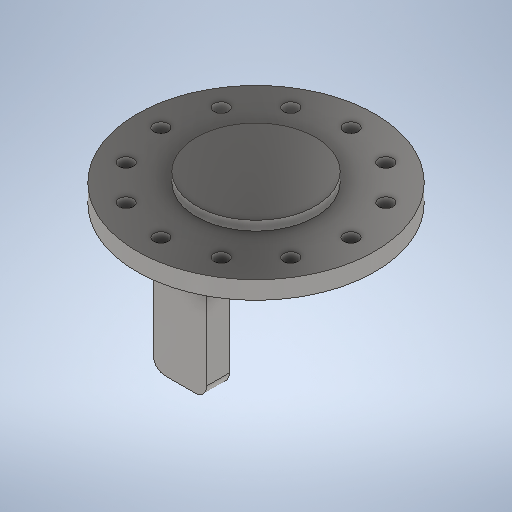
# Autodesk Inventor part: EndEffector
Saved by Autodesk Inventor 2025.1 (Build 291241000, 241)
## iProperties
Created: 2025-01-29
Part Number: EndEffector
Material: Steel, High Strength, Low Alloy
Document SubType Name: Modeling
Designer: yovan
Mass: 4767.32 g
Surface Area: 922.718 cm^2
Volume: 607.302 cm^3
Density: 7.85 g/cm^3
Appearance: Steel - Polished
Author: yovan
Autodesk Inventor part; units mm, degrees
ref_plane "YZ Plane" through (0, 0, 0) normal (1, 0, 0) x (0, 1, 0)
ref_plane "XZ Plane" through (0, 0, 0) normal (0, 1, 0) x (-1, 0, 0)
ref_plane "XY Plane" through (0, 0, 0) normal (0, 0, 1) x (1, 0, 0)
sketch "Sketch3" plane through (0, 0, 0) normal (0, 1, 0) x (-1, 0, 0)
  circle A0 centre (0, 0) radius 100
  dimension "d10" = 200
  constraints: 1 centre point, 1 coincident
  measures "d10" diameter of A0
extrude "Extrusion3" add sketch "Sketch3" along normal blind 15
sketch "Sketch5" plane through (0, 15, 0) normal (0, 1, 0) x (1, 0, 0)
  circle A0 centre (0, 0) radius 80
  circle A1 centre (0, 80) radius 6
  circle A2 centre (-40, 69.282) radius 6
  circle A3 centre (-69.282, 40) radius 6
  circle A4 centre (-80, 0) radius 6
  circle A5 centre (-69.282, -40) radius 6
  circle A6 centre (-40, -69.282) radius 6
  circle A7 centre (0, -80) radius 6
  circle A8 centre (40, -69.282) radius 6
  circle A9 centre (69.282, -40) radius 6
  circle A10 centre (80, 0) radius 6
  circle A11 centre (69.282, 40) radius 6
  circle A12 centre (40, 69.282) radius 6
  circle A13 centre (0, 0) radius 50
  dimension "d13" = 160
  dimension "d14" = 12
  dimension "d17" = 360
  dimension "d19" = 100
  constraints: 13 centre point, 2 coincident, 1 vertical alignment, 27 other
  measures "d14" diameter of A1
  measures "d19" diameter of A13
extrude "Extrusion4" cut sketch "Sketch5" against normal blind 20 contours A0 A10 | A0 A10 | A11 A0 | A0 A11 | A9 A0 | A0 A9 | A12 A0 | A0 A12 | A8 A0 | A0 A8 | A1 A0 | A0 A1 | A7 A0 | A0 A7 | A2 A0 | A0 A2 | A6 A0 | A0 A6 | A3 A0 | A0 A3 | A5 A0 | A0 A5 | A4 A0 | A0 A4
extrude "Extrusion5" add sketch "Sketch5" along normal blind 8 contours A13
sketch "Sketch6" plane through (0, 0, 0) normal (0, -1, 0) x (1, 0, 0)
  circle A0 centre (0, 80) radius 6 projected
  line L0 (22.5, 64) -> (-22.5, 64)
  line L1 (-22.5, 64) -> (-22.5, 44)
  line L2 (-22.5, 44) -> (22.5, 44)
  line L3 (22.5, 44) -> (22.5, 64)
  dimension "d28" = 45
  dimension "d29" = 20
  constraints: 8 end point, 2 parallel, 1 horizontal, 1 perpendicular
  measures "d28" distance of L2.end L1.end
  measures "d29" distance of L1.end L0.end
extrude "Extrusion6" add sketch "Sketch6" along normal blind 100 contours L3 L2 L1 L0
fillet "Fillet1" radius 10 1 edges at (-22.5, -100, 54)
fillet "Fillet2" radius 10 1 edges at (22.5, -100, 54)
sketch "Sketch8" plane through (22.5, 0, 44) normal (0, 0, -1) x (-1, 0, 0)
  line L0 (22.5, 0) -> (22.5, -40)
  line L1 (22.5, -40) -> (22.5, -75)
  circle A0 centre (22.5, -75) radius 7.5
  circle A1 centre (22.5, -40) radius 7.5
  point P0 (22.5, -32.5)
  point P1 (22.5, -47.5)
  dimension "d37" = 40
  dimension "d38" = 35
  dimension "d39" = 15
  dimension "d40" = 15
  constraints: 4 end point, 2 centre point, 2 coincident, 2 vertical
  measures "d37" distance of L0.start L0.end
  measures "d38" distance of L0.end L1.end
  measures "d39" diameter of A0
  measures "d40" diameter of A1
extrude "Extrusion7" add sketch "Sketch8" along normal blind 10
fillet "Face Fillet1" radius 10 1 edges at (0, 0, 44)
fillet "Fillet3" radius 1 7 edges at (19.5711, -97.0711, 44) (0, -100, 44) (-19.5711, -97.0711, 44) (-22.5, -50, 44) (-22.5, -2.9289, 41.0711) (22.5, -2.9289, 41.0711) (22.5, -50, 44)
body "Solid2"
